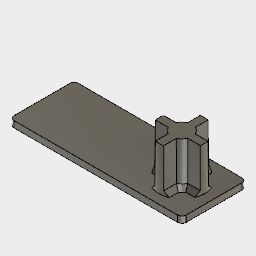
z-drag-chain-plate (Autodesk Fusion 360 design; units mm, degrees)
Autodesk Fusion 360 part; units mm, degrees
sketch "Sketch2" plane through (0, 0, 0) normal (0, 0, 1) x (1, 0, 0)
  line L0 (-65, -15) -> (15, -15)
  line L1 (15, -15) -> (15, 15)
  line L2 (15, 15) -> (-65, 15)
  line L3 (-65, 15) -> (-65, -15)
  dimension "d8" = 30
  dimension "d24" = 80
  measures "d8" distance of L0.start L2.end
  measures "d24" distance of L1.end L2.end
extrude "Extrude1" add sketch "Sketch2" along normal blind 3
sketch "Sketch1" plane through (0, 0, 3) normal (0, 0, 1) x (1, 0, 0)
  circle A0 centre (0, 0) radius 12.5 construction
  circle A1 centre (0, 0) radius 10.7
  circle A2 centre (0, 0) radius 5
  line L0 (-2.0135, 4.5767) -> (-2.0252, 10.5066)
  line L1 (2.0251, 10.5066) -> (2.0135, 4.5766)
  line L2 (4.6132, 1.9281) -> (10.5228, 1.9392)
  line L3 (10.5228, -1.9392) -> (4.6132, -1.9282)
  line L4 (-2.0678, -4.5524) -> (-2.0798, -10.4959)
  line L5 (2.0798, -10.4959) -> (2.0677, -4.5524)
  line L6 (-4.5484, -2.0767) -> (-10.4941, -2.0888)
  line L7 (-10.4941, 2.0888) -> (-4.5484, 2.0767)
  line L8 (-65, 15) -> (-65, -15)
  line L9 (-65, -15) -> (15, -15)
  line L10 (15, -15) -> (15, 15)
  line L11 (15, 15) -> (-65, 15)
  dimension "d23" = 21.4
  measures "d23" diameter of A1
fillet "Fillet1" radius 2 1 edges at (15, -15, 1.5)
fillet "Fillet2" radius 2 1 edges at (-65, -15, 1.5)
fillet "Fillet3" radius 2 1 edges at (15, 15, 1.5)
fillet "Fillet4" radius 2 1 edges at (-65, 15, 1.5)
extrude "Extrude3" add sketch "Sketch1" along normal blind 20 draft -0.5 contours A1 A2 L2 L3 | A1 A2 L0 L1 | A2 | A1 A2 L4 L5 | A1 A2 L6 L7
chamfer "Chamfer1" distance 2 angle 45 12 edges at (2.0737, -7.5242, 3) (3.5889, -3.4813, 3) (7.568, -1.9337, 3) (7.568, 1.9337, 3) (3.5682, 3.5025, 3) (2.0193, 7.5416, 3) (-2.0193, 7.5416, 3) (-3.511, 3.5599, 3) (-7.5212, 2.0828, 3) (-7.5212, -2.0828, 3) (-3.5321, -3.539, 3) (-2.0738, -7.5242, 3)
equation "OD = 25 mm"
equation "ID = 21 mm"
equation "WallThickness = 2 mm"
equation "Length = 80 mm"
equation "d8 = OD + ( 2 * 2 ) * 1 mm + 1 mm"
equation "d10 = WallThickness + 1 mm"
equation "d23 = ID + 0.4 mm"
equation "d24 = Length"
named bodies: "z-drag-chain-plate"
